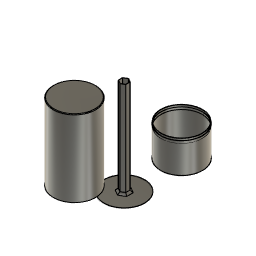
lamp v9 (Autodesk Fusion 360 design; units mm, degrees)
Autodesk Fusion 360 part; units mm, degrees
sketch "Sketch1" plane through (0, 0, 0) normal (0, 0, 1) x (1, 0, 0)
  circle A0 centre (0, 0) radius 55
  circle A1 centre (0, 0) radius 54.35
  circle A2 centre (0, 0) radius 53.35
  dimension "d1" = 110
  dimension "d12" = -0.65
  dimension "d13" = -1.65
  constraint coincident A0.centre A1.centre
  measures "d1" diameter of A0
extrude "Extrude8" add sketch "Sketch1" against normal blind 80 contours A0 | A1 | A2 makes body 1
shell "Shell3" thickness 1.2 removed faces 1 at (-30.9293, -6.6809, 0) on bodies 1
extrude "Extrude9" add sketch "Sketch1" along normal blind 5 contours A1 bodies 1
fillet "Fillet7" radius 43.25 1 edges at (-50.1592, 19.4549, 0) on bodies 1
fillet "Fillet8" radius 1.5 1 edges at (-51.278, 19.8888, -80) on bodies 1
sketch "Sketch7" plane through (0, 0, 0) normal (0, 1, 0) x (1, 0, 0)
  line L0 (0, 0) -> (0, 74)
  line L1 (-6, 76) -> (6, 76)
  line L2 (6, 76) -> (6, 72)
  line L3 (6, 72) -> (-6, 72)
  line L4 (-6, 72) -> (-6, 76)
  line L5 (-6, 76) -> (6, 72) construction
  line L6 (6, 76) -> (-6, 72) construction
  point P0 (0, 74)
  dimension "d54" = 12
  dimension "d55" = 4
  constraint coincident L0.start origin
  constraint vertical L0
  constraint horizontal L1
  constraint perpendicular L1 L2
  constraint parallel L1 L3
  constraint parallel L2 L4
  constraint coincident L5 P0
  constraint coincident L6 P0
  constraint coincident P0 L0.end
  measures "d54" distance of L2.end L3.end
  measures "d55" distance of L1.end L2.end
extrude "Extrude10" cut sketch "Sketch7" along normal blind 100 bodies 1
extrude "Extrude11" add sketch "Sketch1" along normal blind 200 separate body contours A0 | A1 | A2 makes body 2
fillet "Fillet9" radius 1.5 1 edges at (-51.278, -19.8888, 200) on bodies 2
sketch "Sketch8" plane through (0, 0, -78.8) normal (0, 0, 1) x (-1, 0, 0)
  circle A0 centre (0, 0) radius 53.8
  line L0 (-10, -5.7735) -> (0, -11.547)
  line L1 (0, -11.547) -> (10, -5.7735)
  line L2 (10, -5.7735) -> (10, 5.7735)
  line L3 (10, 5.7735) -> (0, 11.547)
  line L4 (0, 11.547) -> (-10, 5.7735)
  line L5 (-10, 5.7735) -> (-10, -5.7735)
  line L6 (0, 10.8542) -> (-9.4, 5.4271)
  line L7 (-9.4, 5.4271) -> (-9.4, -5.4271)
  line L8 (-9.4, -5.4271) -> (0, -10.8542)
  line L9 (0, -10.8542) -> (9.4, -5.4271)
  line L10 (9.4, -5.4271) -> (9.4, 5.4271)
  line L11 (9.4, 5.4271) -> (0, 10.8542)
  circle A1 centre (0, 0) radius 53.1
  line L12 (0, 10.3923) -> (-9, 5.1962)
  line L13 (-9, 5.1962) -> (-9, -5.1962)
  line L14 (-9, -5.1962) -> (0, -10.3923)
  line L15 (0, -10.3923) -> (9, -5.1962)
  line L16 (9, -5.1962) -> (9, 5.1962)
  line L17 (9, 5.1962) -> (0, 10.3923)
  dimension "d62" = -0.6
  dimension "d65" = -0.7
  dimension "d72" = -1
  constraint coincident A0.centre A1.centre
extrude "Extrude12" add sketch "Sketch8" along normal blind 250 separate body contours L0 L1 L2 L3 L4 L5 makes body 3
extrude "Extrude13" add sketch "Sketch8" along normal blind 0.6 contours A1 bodies 3
fillet "Fillet10" radius 5 tangency weight 0.1 6 edges at (-5, -8.6603, -78.2) (5, -8.6603, -78.2) (10, 0, -78.2) (5, 8.6603, -78.2) (-5, 8.6603, -78.2) (-10, 0, -78.2) on bodies 3
extrude "Extrude14" add sketch "Sketch8" along normal blind 0.6 contours L6 L7 L8 L9 L10 L11 | L12 L13 L14 L15 L16 L17 bodies 3
move_face "MoveFace1" to x (1, 0, 0) y (0, 1, 0) z (0, 0, 1) at (0, -130, 0) 1 faces at (-54.7267, 5.4762, 132.3333) on bodies 2
move_body "Move3" bodies 1 to x (1, 0, 0) y (0, 1, 0) z (0, 0, 1) at (0, 150, 0)
named bodies: "Bottom", "Top", "Center"
